nixal_reprap4040_psuClamp1 (Autodesk Fusion 360 design; units mm, degrees)
Autodesk Fusion 360 part; units mm, degrees
sketch "Sketch1" plane through (0, 0, 0) normal (0, 1, 0) x (1, 0, 0)
  line L0 (0, 0) -> (150, 0)
  line L1 (150, 0) -> (150, 25)
  line L2 (150, 25) -> (0, 25)
  line L3 (0, 25) -> (0, 0)
  line L4 (0, 25) -> (150, 25)
  line L5 (150, 25) -> (150, 30)
  line L6 (150, 30) -> (0, 30)
  line L7 (0, 30) -> (0, 25)
  circle A0 centre (35, 12.5) radius 4
  circle A1 centre (115, 12.5) radius 4
  circle A2 centre (35, 12.5) radius 7.5
  circle A3 centre (115, 12.5) radius 7.5
  dimension "d1" = 25
  dimension "d2" = 8
  dimension "d3" = 8
  dimension "d4" = 35
  dimension "d5" = 35
  dimension "d6" = 15
  dimension "d7" = 15
  constraint horizontal L0
  constraint vertical L1
  constraint horizontal L2
  constraint vertical L3
  constraint coincident L0.start L3.end
  constraint horizontal L4
  constraint vertical L5
  constraint horizontal L6
  constraint vertical L7
  constraint concentric A0 A2
  constraint concentric A1 A3
  measures "d2" diameter of A0
  measures "d3" diameter of A1
  measures "d6" diameter of A2
  measures "d7" diameter of A3
extrude "Extrude1" add sketch "Sketch1" along normal blind 4 contours L0 L1 L2 L3 L4 | A2 | A3 makes body 1
extrude "Extrude2" add sketch "Sketch1" along normal blind 0 and the other way blind -6 separate body contours A2 | A3 makes body 2 at (42.4907, 2, -12.1262) makes body 3 at (122.4907, 2, -12.1262)
extrude "Extrude3" add sketch "Sketch1" along normal blind 24 contours L2 L4 L5 L6 L7 bodies 1
sketch "Sketch2" plane through (0, 0, -30) normal (0, 0, -1) x (-1, 0, 0)
  line L0 (-150, 0) -> (0, 0)
  line L1 (0, 0) -> (0, 24)
  line L2 (0, 24) -> (-150, 24)
  line L3 (-150, 24) -> (-150, 0)
  line L4 (-143.5, 24) -> (-143.5, 0)
  circle A0 centre (-143.5, 18.5) radius 2
  line L5 (-6.5, 24) -> (-6.5, 0)
  circle A1 centre (-6.5, 18.5) radius 2
  circle A2 centre (-143.5, 18.5) radius 4.5
  circle A3 centre (-6.5, 18.5) radius 4.5
  dimension "d15" = 6.5
  dimension "d16" = 4
  dimension "d17" = 18.5
  dimension "d18" = 6.5
  dimension "d19" = 4
  dimension "d20" = 9
  dimension "d21" = 9
  constraint coincident L2 L0.end
  constraint coincident L0 L1.start
  constraint perpendicular L0 L4
  constraint coincident L4 L0.end
  constraint perpendicular L2 L5
  constraint coincident L5 L0.end
  constraint concentric A0 A2
  constraint concentric A1 A3
  measures "d15" distance of L3 L4
  measures "d16" diameter of A0
  measures "d18" distance of L1 L5
  measures "d19" diameter of A1
  measures "d20" diameter of A2
  measures "d21" diameter of A3
extrude "Extrude4" cut sketch "Sketch2" against normal blind 10 contours L4 A0 | L4 A0 | L5 A1 | L5 A1 bodies 1
extrude "Extrude5" cut sketch "Sketch2" along normal blind -10 and the other way blind 2 contours L4 A0 A2 | L4 A0 A2 | L5 A1 A3 | L5 A1 A3 bodies 1
